Servo Dynamixel XL320 (Autodesk Fusion 360 design; units mm, degrees)
Autodesk Fusion 360 part; units mm, degrees
note: some values were not read from the file. Chosen so that the rebuilt part matches the saved one: a direction.
sketch "Sketch1" plane through (0, 0, 0) normal (0, 0, 1) x (1, 0, 0)
  line L0 (12, -18) -> (-12, -18)
  line L1 (-12, -18) -> (-12, 18)
  line L2 (-12, 18) -> (12, 18)
  line L3 (12, 18) -> (12, -18)
  line L4 (12, -18) -> (-12, 18) construction
  line L5 (-12, -18) -> (12, 18) construction
  dimension "d1" = 36
  dimension "d2" = 24
  constraint perpendicular L0 L1
  constraint parallel L0 L2
  constraint parallel L1 L3
  constraint horizontal L0
  constraint coincident L4 origin
  constraint coincident L5 origin
  measures "d1" distance of L0.end L1.end
  measures "d2" distance of L1.end L2.end
  measures "d13" distance of L0.start
extrude "Extrude1" add sketch "Sketch1" along normal blind 24
chamfer "Chamfer1" distance 4 angle 45 4 edges at (12, -18, 12) (12, 18, 12) (-12, -18, 12) (-12, 18, 12)
sketch "Sketch2" plane through (0, 0, 24) normal (0, 0, 1) x (-1, 0, 0)
  line L0 (8, -18) -> (12, -14)
  line L1 (12, -14) -> (12, 14)
  line L2 (12, 14) -> (8, 18)
  line L3 (8, 18) -> (-8, 18)
  line L4 (-8, 18) -> (-12, 14)
  line L5 (-12, 14) -> (-12, -14)
  line L6 (-12, -14) -> (-8, -18)
  line L7 (-8, -18) -> (8, -18)
  circle A0 centre (0, -9) radius 9
  circle A1 centre (0, -9) radius 6 construction
  line L8 (0, 0) -> (0, -18) construction
  circle A2 centre (0, -15) radius 1.75
  circle A3 centre (6, -9) radius 1.75
  circle A4 centre (0, -3) radius 1.75
  circle A5 centre (-6, -9) radius 1.75
  dimension "d6" = 18
  dimension "d7" = 12
  dimension "d8" = 3.5
  dimension "d10" = 360
  constraint concentric A0 A1
  constraint coincident L8.start origin
  constraint midpoint L7 L8.end
  constraint coincident A0.centre L8
  constraint midpoint A0.centre L8
  constraint coincident A1 A2.centre
  constraint coincident L8 A2.centre
  measures "d6" diameter of A0
  measures "d7" diameter of A1
  measures "d8" diameter of A2
extrude "Extrude2" add sketch "Sketch2" along normal blind 3 contours A0
sketch "Sketch3" plane through (0, -18, 0) normal (0, -1, 0) x (1, 0, 0)
  line L0 (-8, 24) -> (-8, 0)
  line L1 (-8, 0) -> (8, 0)
  line L2 (8, 0) -> (8, 24)
  line L3 (8, 24) -> (-8, 24)
  line L4 (-12, 0) -> (12, 0)
  line L5 (12, 0) -> (12, 24)
  line L6 (12, 24) -> (-12, 24)
  line L7 (-12, 24) -> (-12, 0)
  line L8 (-12, 21) -> (12, 21)
  line L9 (-12, 3) -> (12, 3)
  point P0 (-12, 24)
  point P1 (12, 24)
  point P2 (12, 0)
  point P3 (-12, 0)
  dimension "d13" = 3
  dimension "d14" = 3
  constraint horizontal L4
  constraint vertical L5
  constraint horizontal L6
  constraint vertical L7
  constraint coincident P1 L5.end
  constraint coincident P3 L4.start
  constraint coincident L7 L8.start
  constraint coincident L5 L8.end
  constraint perpendicular L5 L8
  constraint coincident L7 L9.start
  constraint coincident L5 L9.end
  constraint perpendicular L5 L9
  measures "d13" distance of L4 L9
  measures "d14" distance of L6 L8
extrude "Extrude3" cut sketch "Sketch3" against normal blind 4.5 contours L0 L2 L8 L9 | L0 L7 L8 L9 | L2 L5 L8 L9
sketch "Sketch5" plane through (0, 0, 24) normal (0, 0, 1) x (-1, 0, 0)
  line L0 (8, -18) -> (12, -14)
  line L1 (12, -14) -> (12, 14)
  line L2 (12, 14) -> (8, 18)
  line L3 (8, 18) -> (-8, 18)
  line L4 (-8, 18) -> (-12, 14)
  line L5 (-12, 14) -> (-12, -14)
  line L6 (-12, -14) -> (-8, -18)
  line L7 (-8, -18) -> (0, -18)
  circle A0 centre (0, -9) radius 9
  line L8 (0, -18) -> (8, -18)
  line L9 (12, 14) -> (-12, 14) construction
  line L10 (0, 14) -> (0, 18) construction
  line L11 (10, 16) -> (-10, 16) construction
  circle A1 centre (0, 16) radius 1.7
  circle A2 centre (-6, 16) radius 1.7
  circle A3 centre (6, 16) radius 1.7
  dimension "d17" = 3.4
  dimension "d20" = 6
  dimension "d21" = 0
  constraint coincident L1.end L2.start
  constraint coincident L4.end L5.start
  constraint midpoint L9 L10.start
  constraint midpoint L3 L10.end
  constraint midpoint L2 L11.start
  constraint midpoint L4 L11.end
  constraint midpoint L11 A1.centre
  measures "d17" diameter of A1
extrude "Extrude4" cut sketch "Sketch5" against normal through all contours A1 | A2 | A3
